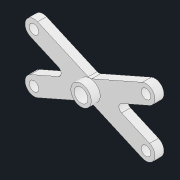
# Autodesk Inventor part: base21
Saved by Autodesk Inventor 2021 (Build 250183000, 183)
## iProperties
Created: 2021-08-08
Part Number: base21
Material: ABS プラスチック
Document SubType Name: Modeling
Designer: yuta0
Density: 1.06 g/cm^3
Appearance: 滑らか - 白
Mass: 4.76056 g
Surface Area: 34.5583 cm^2
Volume: 4.49109 cm^3
在庫数: 0.0
購入先: 印刷
Author: yuta0
Autodesk Inventor part; units mm, degrees
ref_plane "YZ Plane" through (0, 0, 0) normal (1, 0, 0) x (0, 1, 0)
ref_plane "XZ Plane" through (0, 0, 0) normal (0, 1, 0) x (-1, 0, 0)
ref_plane "XY Plane" through (0, 0, 0) normal (0, 0, 1) x (1, 0, 0)
sketch "スケッチ1" plane through (0, 0, 0) normal (0, 0, 1) x (1, 0, 0)
  line L0 (-25, -11) -> (25, -11) construction
  line L1 (25, -11) -> (25, 11) construction
  line L2 (25, 11) -> (-25, 11) construction
  line L3 (-25, 11) -> (-25, -11) construction
  line L4 (-25, -11) -> (25, 11) construction
  line L5 (25, -11) -> (-25, 11) construction
  line L6 (25, -11) -> (-25, 11) construction
  line L7 (26.611, -7.3387) -> (-23.389, 14.6613)
  line L8 (-26.611, 7.3387) -> (23.389, -14.6613)
  arc A0 (23.389, -14.6613) -> (26.611, -7.3387) centre (25, -11) ccw
  arc A1 (-23.389, 14.6613) -> (-26.611, 7.3387) centre (-25, 11) ccw
  line L9 (-25, -11) -> (25, 11) construction
  line L10 (-23.389, -14.6613) -> (26.611, 7.3387)
  line L11 (23.389, 14.6613) -> (-26.611, -7.3387)
  arc A2 (-26.611, -7.3387) -> (-23.389, -14.6613) centre (-25, -11) ccw
  arc A3 (26.611, 7.3387) -> (23.389, 14.6613) centre (25, 11) ccw
  point P0 (0, 0)
  point P1 (0, 4.3701)
  point P2 (-9.932, 0)
  point P3 (0, -4.3701)
  point P4 (9.932, 0)
  dimension "d0" = 50
  dimension "d1" = 22
  dimension "d2" = 8
  dimension "d3" = 8
  constraints: 28 end point, 8 point on circle, 8 tangent, 5 equal length, 4 centre point, 4 midpoint, 1 horizontal, 1 perpendicular
  measures "d0" distance of L2.end L1.end
  measures "d1" distance of L1.end L0.end
  measures "d2" diameter of A1
  measures "d3" diameter of A3
extrude "押し出し1" add sketch "スケッチ1" along normal blind 4
fillet "フィレット1" radius 2 4 edges at (0, -4.3701, 2) (-9.932, 0, 2) (0, 4.3701, 2) (9.932, 0, 2)
sketch "スケッチ2" plane through (0, 0, 4) normal (0, 0, 1) x (1, 0, 0)
  arc A0 (-23.389, 14.6613) -> (-26.611, 7.3387) centre (-25, 11) ccw projected
  arc A1 (-26.611, -7.3387) -> (-23.389, -14.6613) centre (-25, -11) ccw projected
  arc A2 (23.389, -14.6613) -> (26.611, -7.3387) centre (25, -11) ccw projected
  arc A3 (26.611, 7.3387) -> (23.389, 14.6613) centre (25, 11) ccw projected
  point P0 (0, 0)
  point P1 (-28.3993, 7.3333)
  point P2 (-28.3993, -7.3333)
  point P3 (28.3993, -7.3333)
  point P4 (28.3993, 7.3333)
hole "穴1" at (-25, 11, 4) at (25, 11, 4) at (25, -11, 4) at (-25, -11, 4) direction (0, 0, -1) diameter 4.3 end through all clearance for "Flat Head Machine Screw" size "M4" standard "Ansi Metric M Profile"
sketch "スケッチ3" plane through (0, 0, 4) normal (0, 0, 1) x (1, 0, 0)
  circle A0 centre (0, 0) radius 3.1
  dimension "d15" = 6.2
  constraints: 1 centre point, 1 coincident
  measures "d15" diameter of A0
extrude "押し出し2" cut sketch "スケッチ3" against normal blind 8
sketch "スケッチ4" plane through (0, 0, 4) normal (0, 0, 1) x (1, 0, 0)
  circle A0 centre (0, 0) radius 3.1 projected
  circle A1 centre (0, 0) radius 4.5551
  arc A2 (-0.8055, 4.7245) -> (0.8055, 4.7245) centre (0, 6.5551) ccw projected
  constraints: 1 centre point, 1 tangent
extrude "押し出し3" add sketch "スケッチ4" along normal blind 4
